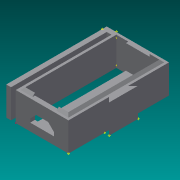
# Autodesk Inventor part: nano_enclosure_modular
Saved by Autodesk Inventor 2015 (Build 190159000, 159)
## iProperties
Created: 2015-02-05
Part Number: nano_enclosure_modular
Material: Generic
Document SubType Name: Modeling
Designer: Jeff
Density: 1 g/cm^3
Appearance: Default
Author: Jeff
Autodesk Inventor part; units mm, degrees
ref_plane "YZ Plane" through (0, 0, 0) normal (1, 0, 0) x (0, 1, 0)
ref_plane "XZ Plane" through (0, 0, 0) normal (0, 1, 0) x (-1, 0, 0)
ref_plane "XY Plane" through (0, 0, 0) normal (0, 0, 1) x (1, 0, 0)
sketch "Sketch1" plane through (0, 0, 0) normal (0, 1, 0) x (-1, 0, 0)
  line L0 (0, 0) -> (27.94, 0)
  line L1 (27.94, 0) -> (27.94, -53.34)
  line L2 (27.94, -53.34) -> (0, -53.34)
  line L3 (0, -53.34) -> (0, 0)
  dimension "d0" = 27.94
  dimension "d1" = 53.34
  constraints: 8 end point, 2 parallel, 1 horizontal, 1 perpendicular
  measures "d0" distance of L1.end L2.end
  measures "d1" distance of L0.end L1.end
extrude "Extrusion1" add sketch "Sketch1" along normal blind 15.24
shell "Shell1" thickness 2.54 removed faces 1 at (-9.3133, 15.24, -17.78)
sketch "Sketch3" plane through (-27.94, 0, 0) normal (0, 0, 1) x (1, 0, 0)
  line L0 (20.32, 4.064) -> (7.62, 4.064)
  line L1 (7.62, 4.064) -> (7.62, 9.144)
  line L2 (7.62, 9.144) -> (20.32, 9.144)
  line L3 (20.32, 9.144) -> (20.32, 4.064)
  point P0 (27.94, 0)
  dimension "d20" = 4.064
  dimension "d21" = 12.7
  dimension "d22" = 5.08
  dimension "d23" = 7.62
  constraints: 8 end point, 2 parallel, 1 horizontal, 1 perpendicular
  measures "d20" distance from line of point (27.94, 0) L0
  measures "d21" distance of L1.end L2.end
  measures "d22" distance of L2.end L0.start
  measures "d23" distance from line of point (27.94, 0) L3
extrude "Extrusion3" cut sketch "Sketch3" against normal blind 2.54
chamfer "Chamfer1" distance 3.175 angle 45 2 edges at (-20.32, 9.144, -1.27) (-7.62, 9.144, -1.27)
sketch "Sketch5" plane through (-25.4, 2.54, -2.54) normal (0, 1, 0) x (1, 0, 0)
  line L0 (0, 0) -> (5.08, 0)
  line L1 (5.08, 0) -> (5.08, 48.26)
  line L2 (5.08, 48.26) -> (0, 48.26)
  line L3 (0, 48.26) -> (0, 0)
  line L4 (0, 48.26) -> (22.86, 48.26) projected
  line L5 (22.86, 0) -> (17.78, 0)
  line L6 (17.78, 0) -> (17.78, 48.26)
  line L7 (17.78, 48.26) -> (22.86, 48.26)
  line L8 (22.86, 48.26) -> (22.86, 0)
  point P0 (25.4, -2.54)
  dimension "d29" = 5.08
  dimension "d30" = 5.08
  constraints: 16 end point, 4 parallel, 2 coincident, 2 horizontal, 2 perpendicular, 1 point on line
  measures "d29" distance between parallel lines of L1 L3
  measures "d30" distance between parallel lines of L8 L6
extrude "Extrusion4" cut sketch "Sketch5" against normal blind 2.54
sketch "Sketch6" plane through (-27.94, 0, -53.34) normal (-1, 0, 0) x (0, 0, 1)
  point P0 (53.34, 0)
sketch "Sketch7" plane through (-27.94, 0, -53.34) normal (-1, 0, 0) x (0, 0, 1)
  line L0 (2.54, 15.24) -> (50.8, 15.24) projected
  line L1 (0, 0) -> (2.54, 0)
  line L2 (2.54, 0) -> (2.54, 15.24)
  line L3 (2.54, 15.24) -> (0, 15.24)
  line L4 (0, 15.24) -> (0, 0)
  point P0 (53.34, 0)
  dimension "d33" = 2.54
  constraints: 8 end point, 2 parallel, 1 coincident, 1 horizontal, 1 perpendicular, 1 point on line
  measures "d33" distance between parallel lines of L4 L2
extrude "Extrusion5" add sketch "Sketch7" along normal blind 5.08
sketch "Sketch8" plane through (-27.94, 0, -50.8) normal (0, 0, 1) x (1, 0, 0)
  line L0 (-5.08, 15.24) -> (-2.54, 15.24)
  line L1 (-2.54, 15.24) -> (-2.54, 0)
  line L2 (-2.54, 0) -> (-5.08, 0)
  line L3 (-5.08, 0) -> (-5.08, 15.24)
  point P0 (27.94, 0)
  dimension "d36" = 2.54
  constraints: 8 end point, 2 coincident, 2 parallel, 1 horizontal, 1 perpendicular
  measures "d36" distance between parallel lines of L3 L1
extrude "Extrusion6" add sketch "Sketch8" along normal up to surface (50.8 mm away)
chamfer "Chamfer2" distance 1.27 angle 45 6 edges at (-2.54, 0, -26.67) (-5.08, 0, -2.54) (-5.08, 0, -50.8) (-22.86, 0, -2.54) (-25.4, 0, -26.67) (-22.86, 0, -50.8)
sketch "Sketch11" plane through (0, 15.24, 0) normal (0, 1, 0) x (1, 0, 0)
  line L0 (-26.67, 52.07) -> (-17.78, 52.07)
  line L1 (-20.32, 1.27) -> (-26.67, 1.27)
  line L2 (-26.67, 1.27) -> (-26.67, 52.07)
  line L3 (-25.4, 2.54) -> (-25.4, 50.8) projected
  line L4 (-2.54, 2.54) -> (-25.4, 2.54) projected
  line L5 (-25.4, 50.8) -> (-2.54, 50.8) projected
  line L6 (-1.27, 52.07) -> (-7.62, 52.07)
  line L7 (-7.62, 1.27) -> (-1.27, 1.27)
  line L8 (-1.27, 1.27) -> (-1.27, 52.07)
  line L9 (-2.54, 50.8) -> (-2.54, 2.54) projected
  line L10 (-7.62, 52.07) -> (-1.27, 52.07)
  line L11 (-1.27, 52.07) -> (-1.27, 50.8)
  line L12 (-1.27, 50.8) -> (-7.62, 50.8)
  line L13 (-7.62, 50.8) -> (-7.62, 52.07)
  line L14 (-2.54, 50.8) -> (-1.27, 50.8)
  line L15 (-1.27, 50.8) -> (-1.27, 1.27)
  line L16 (-1.27, 1.27) -> (-2.54, 1.27)
  line L17 (-2.54, 1.27) -> (-2.54, 50.8)
  line L18 (-2.54, 2.54) -> (-7.62, 2.54)
  line L19 (-7.62, 2.54) -> (-7.62, 1.27)
  line L20 (-7.62, 1.27) -> (-2.54, 1.27)
  line L21 (-2.54, 1.27) -> (-2.54, 2.54)
  line L22 (-26.67, 52.07) -> (-20.32, 52.07)
  line L23 (-20.32, 52.07) -> (-20.32, 50.8)
  line L24 (-20.32, 50.8) -> (-26.67, 50.8)
  line L25 (-26.67, 50.8) -> (-26.67, 52.07)
  line L26 (-25.4, 50.8) -> (-26.67, 50.8)
  line L27 (-26.67, 50.8) -> (-26.67, 1.27)
  line L28 (-26.67, 1.27) -> (-25.4, 1.27)
  line L29 (-25.4, 1.27) -> (-25.4, 50.8)
  line L30 (-25.4, 2.54) -> (-20.32, 2.54)
  line L31 (-20.32, 2.54) -> (-20.32, 1.27)
  line L32 (-20.32, 1.27) -> (-25.4, 1.27)
  line L33 (-25.4, 1.27) -> (-25.4, 2.54)
  point P0 (0, 0)
  dimension "d50" = 1.27
  dimension "d51" = 1.27
  dimension "d52" = 1.27
  dimension "d55" = 1.27
  dimension "d57" = 1.27
  dimension "d58" = 5.08
  dimension "d59" = 48.26
  dimension "d60" = 6.35
  dimension "d61" = 6.35
  constraints: 60 end point, 14 parallel, 8 horizontal, 6 perpendicular, 2 point on line
  measures "d50" distance between parallel lines of L2 L3
  measures "d51" distance between parallel lines of L1 L4
  measures "d52" distance between parallel lines of L5 L0
  measures "d55" distance between parallel lines of L8 L9
  measures "d57" distance between parallel lines of L5 L6
  measures "d58" distance between parallel lines of L9 L13
  measures "d59" distance between parallel lines of L12 L4
  measures "d60" distance between parallel lines of L25 L23
  measures "d61" distance between parallel lines of L2 L31
extrude "Extrusion8" add sketch "Sketch11" along normal blind 1.27 contours L0 L23 L5 L24 L2 | L24 L3 L29 L1 L2 | L13 L6 L8 L12 L5 | L29 L4 L31 L1 | L12 L8 L7 L17 L9 | L17 L7 L19 L4
chamfer "Chamfer3" distance 1.27 angle 45 6 edges at (-1.27, 16.51, -26.67) (-4.445, 16.51, -1.27) (-4.445, 16.51, -52.07) (-23.495, 16.51, -52.07) (-26.67, 16.51, -26.67) (-23.495, 16.51, -1.27)
sketch "Sketch12" plane through (0, 0, 0) normal (1, 0, 0) x (0, 0, -1)
  line L0 (52.07, 0) -> (1.27, 0) projected
  line L1 (0, 15.24) -> (53.34, 15.24) projected
  line L2 (19.05, 0) -> (34.29, 0)
  line L3 (34.29, 0) -> (34.29, 15.24)
  line L4 (34.29, 15.24) -> (19.05, 15.24)
  line L5 (19.05, 15.24) -> (19.05, 0)
  line L6 (0, 0) -> (0, 15.24) projected
  line L7 (53.34, 0) -> (53.34, 15.24) projected
  dimension "d67" = 19.05
  dimension "d68" = 19.05
  constraints: 8 end point, 2 parallel, 2 point on line, 1 horizontal, 1 perpendicular
  measures "d67" distance between parallel lines of L6 L5
  measures "d68" distance between parallel lines of L7 L3
extrude "Extrusion9" add sketch "Sketch12" along normal blind 2.54
sketch "Sketch14" plane through (0, 0, 0) normal (0, -1, 0) x (1, 0, 0)
  line L0 (0, -19.05) -> (0, -21.59)
  line L1 (2.54, -19.05) -> (0, -21.59)
  line L2 (0, -34.29) -> (0, -31.75)
  line L3 (0, -31.75) -> (2.54, -34.29)
  line L4 (0, -19.05) -> (2.54, -19.05)
  line L5 (0, -19.05) -> (2.54, -19.05) projected
  line L6 (2.54, -34.29) -> (0, -34.29)
  line L7 (0, -53.34) -> (0, -34.29) projected
  point P0 (0, 0)
  dimension "d71" = 2.54
  dimension "d72" = 2.54
  constraints: 12 end point, 2 vertical, 1 collinear, 1 perpendicular
  measures "d71" distance of L0.start L0.end
  measures "d72" distance of L2.start L2.end
extrude "Extrusion10" cut sketch "Sketch14" against normal blind 25.4
body "Solid1"
